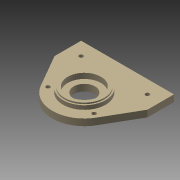
# Autodesk Inventor part: 砂轮轴端盖
Saved by Autodesk Inventor 2015 (Build 190159000, 159)
## iProperties
Created: 2017-05-16
Part Number: 砂轮轴端盖
Material: 常规
Document SubType Name: Modeling
Designer: Administrator
Density: 1 g/cm^3
Appearance: 米色
Author: Administrator
Autodesk Inventor part; units mm, degrees
ref_plane "YZ Plane" through (0, 0, 0) normal (1, 0, 0) x (0, 1, 0)
ref_plane "XZ Plane" through (0, 0, 0) normal (0, 1, 0) x (-1, 0, 0)
ref_plane "XY Plane" through (0, 0, 0) normal (0, 0, 1) x (1, 0, 0)
sketch "草图1" plane through (0, 0, 0) normal (0, 0, 1) x (1, 0, 0)
  circle A0 centre (0, 0) radius 24
  line L0 (-20.7846, -12) -> (-34.9297, 12.5)
  line L1 (-34.9297, 12.5) -> (-34.9297, 32.5)
  line L2 (-34.9297, 32.5) -> (34.9297, 32.5)
  line L3 (34.9297, 32.5) -> (34.9297, 12.5)
  line L4 (34.9297, 12.5) -> (20.7846, -12)
  line L5 (0, 0) -> (0, 15.9109)
  dimension "d0" = 48
  dimension "d1" = 15.9109
  dimension "d2" = 12.5
  dimension "d3" = 20
  dimension "d4" = 150
  constraints: 12 end point, 2 equal length, 2 perpendicular, 2 point on circle, 2 tangent, 2 vertical, 1 centre point, 1 coincident
  measures "d0" diameter of A0
  measures "d1" distance of L5.start L5.end
  measures "d2" vertical distance of point (0, 0) L3.end
  measures "d3" distance of L2.end L3.end
  measures "d4" angle of L3 L4
extrude "拉伸1" add sketch "草图1" along normal blind 5
sketch "草图2" plane through (0, 0, 5) normal (0, 0, 1) x (1, 0, 0)
  circle A0 centre (0, 0) radius 16
  circle A1 centre (0, 0) radius 12.5
  dimension "d7" = 32
  dimension "d8" = 25
  constraints: 2 centre point, 2 coincident
  measures "d7" diameter of A0
  measures "d8" diameter of A1
extrude "拉伸2" add sketch "草图2" along normal blind 4
sketch "草图3" plane through (0, 0, 9) normal (0, 0, 1) x (1, 0, 0)
  circle A0 centre (0, 0) radius 16
  circle A1 centre (0, 0) radius 15
  dimension "d11" = 32
  dimension "d12" = 30
  constraints: 2 centre point, 2 coincident
  measures "d11" diameter of A0
  measures "d12" diameter of A1
extrude "拉伸3" cut sketch "草图3" against normal blind 1
sketch "草图4" plane through (0, 0, 5) normal (0, 0, 1) x (1, 0, 0)
  circle A0 centre (0, 0) radius 8
  dimension "d15" = 16
  constraints: 1 centre point, 1 coincident
  measures "d15" diameter of A0
extrude "拉伸4" cut sketch "草图4" against normal through all
sketch "草图5" plane through (0, 0, 5) normal (0, 0, 1) x (1, 0, 0)
  circle A0 centre (17.3205, -10) radius 1.5
  circle A1 centre (-17.3205, -10) radius 1.5
  circle A2 centre (24.9297, 22.5) radius 1.5
  circle A3 centre (-24.9297, 22.5) radius 1.5
  line L0 (-34.9297, 32.5) -> (-34.9297, 12.5) projected
  line L1 (34.9297, 32.5) -> (-34.9297, 32.5) projected
  line L2 (34.9297, 12.5) -> (34.9297, 32.5) projected
  arc A4 (-17.3205, -10) -> (17.3205, -10) centre (0, 0) ccw
  dimension "d18" = 3
  dimension "d19" = 3
  dimension "d20" = 3
  dimension "d21" = 3
  dimension "d22" = 10
  dimension "d23" = 10
  dimension "d24" = 10
  dimension "d25" = 10
  dimension "d26" = 10
  dimension "d27" = 20
  dimension "d28" = 10
  constraints: 5 centre point, 2 point on circle, 1 coincident
  measures "d18" diameter of A0
  measures "d19" diameter of A1
  measures "d20" diameter of A2
  measures "d21" diameter of A3
  measures "d22" distance from line of L0 A3.centre
  measures "d23" distance from line of L1 A3.centre
  measures "d24" distance from line of L2 A2.centre
  measures "d25" distance from line of L1 A2.centre
  measures "d26" vertical distance of point (0, 0) A1.centre
  measures "d27" radius of A4
  measures "d28" vertical distance of point (0, 0) A0.centre
extrude "拉伸5" cut sketch "草图5" against normal through all
sketch "草图6" plane through (0, 0, 0) normal (0, 0, -1) x (-1, 0, 0)
  circle A0 centre (17.3205, -10) radius 2.5
  circle A1 centre (-17.3205, -10) radius 2.5
  circle A2 centre (24.9297, 22.5) radius 2.5
  circle A3 centre (-24.9297, 22.5) radius 2.5
  circle A4 centre (17.3205, -10) radius 1.5 projected
  circle A5 centre (-17.3205, -10) radius 1.5 projected
  circle A6 centre (-24.9297, 22.5) radius 1.5 projected
  circle A7 centre (24.9297, 22.5) radius 1.5 projected
  point P0 (0, 0)
  dimension "d31" = 5
  dimension "d32" = 5
  dimension "d33" = 5
  dimension "d34" = 5
  constraints: 4 centre point, 4 concentric
  measures "d31" diameter of A0
  measures "d32" diameter of A1
  measures "d33" diameter of A2
  measures "d34" diameter of A3
extrude "拉伸6" cut sketch "草图6" against normal blind 2.5
